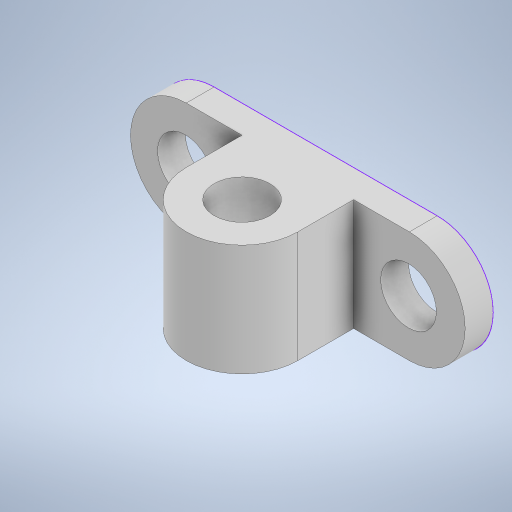
# Autodesk Inventor part: TAREA # 1 LAB DINAMICA
Saved by Autodesk Inventor 2024 (Build 280153000, 153)
## iProperties
Created: 2024-01-27
Part Number: TAREA # 1 LAB DINAMICA
Material: Genérico
Document SubType Name: Modeling
Designer: Eva Sinay
Density: 1 g/cm^3
Appearance: Valor por defecto
Author: Eva Sinay
Autodesk Inventor part; units mm, degrees
ref_plane "YZ Plane" through (0, 0, 0) normal (1, 0, 0) x (0, 1, 0)
ref_plane "XZ Plane" through (0, 0, 0) normal (0, 1, 0) x (-1, 0, 0)
ref_plane "XY Plane" through (0, 0, 0) normal (0, 0, 1) x (1, 0, 0)
sketch "Boceto1" plane through (0, 0, 0) normal (0, 0, 1) x (1, 0, 0)
  line L0 (-40, 20) -> (40, 20)
  line L1 (40, -20) -> (-40, -20)
  circle A0 centre (-40, 0) radius 20
  circle A1 centre (40, 0) radius 20
  line L2 (-20, 20) -> (20, 20)
  line L3 (20, 20) -> (20, -20)
  line L4 (20, -20) -> (-20, -20)
  line L5 (-20, -20) -> (-20, 20)
  point P0 (0, 0)
  constraints: 12 end point, 3 parallel, 2 centre point, 2 horizontal, 1 perpendicular, 1 point on line
extrude "Extrusión1" add sketch "Boceto1" along normal blind 10 contours L0 L5 A0 | A0 | L5 L1 A0 | L0 A1 L3 | A1 | A1 L1 L3
sketch "Boceto2" plane through (0, 0, 0) normal (0, 0, 1) x (1, 0, 0)
  line L0 (20, 20) -> (20, -20) projected
  line L1 (-20, 20) -> (20, 20)
  line L2 (20, 20) -> (20, -20)
  line L3 (20, -20) -> (-20, -20)
  line L4 (-20, -20) -> (-20, 20)
  line L5 (-20, 20) -> (20, -20) construction
  line L6 (20, 20) -> (-20, -20) construction
  point P0 (0, 0)
  constraints: 12 end point, 2 midpoint, 2 parallel, 1 horizontal, 1 perpendicular
extrude "Extrusión2" add sketch "Boceto2" along normal blind 30
sketch "Boceto3" plane through (0, 0, 0) normal (0, 0, -1) x (-1, 0, 0)
  circle A0 centre (-39.6971, 0) radius 10
  circle A1 centre (40.3162, 0) radius 10
  point P0 (0, 0)
  constraints: 2 centre point
extrude "Extrusión3" cut sketch "Boceto3" against normal blind 10
sketch "Boceto4" plane through (-40, -20, 0) normal (0, -1, 0) x (1, 0, 0)
  line L0 (20, 30) -> (60, 30) projected
  circle A0 centre (40, 30) radius 20
  point P0 (40, 0)
  constraints: 1 midpoint, 3 other
extrude "Extrusión4" add sketch "Boceto4" against normal blind 40 contours A0 L0 picked at (46.4729, 31.5954)
sketch "Boceto5" plane through (-40, -20, 0) normal (0, -1, 0) x (1, 0, 0)
  arc A0 (60, 30) -> (20, 30) centre (40, 30) ccw projected
  circle A1 centre (40, 30) radius 10
  point P0 (40, 0)
  dimension "d15" = 20
  constraints: 1 centre point, 1 coincident
  measures "d15" diameter of A1
extrude "Extrusión5" cut sketch "Boceto5" against normal blind 40
